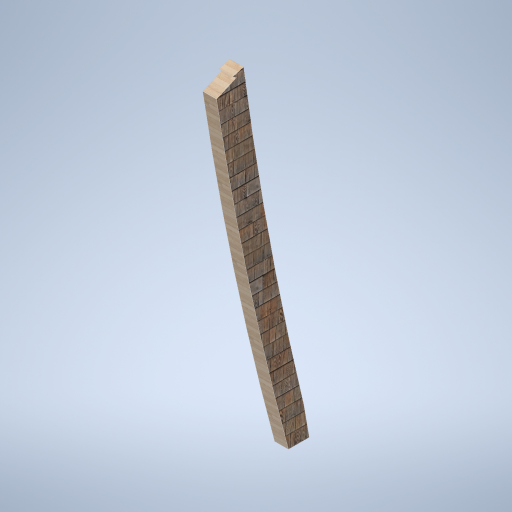
# Autodesk Inventor part: side_curve_beam_02
Saved by Autodesk Inventor 2024.2 (Build 282272000, 272)
## iProperties
Created: 2024-05-24
Part Number: side_curve_beam_02
Material: Wood (Maple)
Document SubType Name: Modeling
Designer: LOSTER_1
Density: 0.67 g/cm^3
Appearance: Natural Maple - Glossy Dark Tint
Author: LOSTER_1
Autodesk Inventor part; units mm, degrees
ref_plane "YZ Plane" through (0, 0, 0) normal (1, 0, 0) x (0, 1, 0)
ref_plane "XZ Plane" through (0, 0, 0) normal (0, 1, 0) x (-1, 0, 0)
ref_plane "XY Plane" through (0, 0, 0) normal (0, 0, 1) x (1, 0, 0)
sketch "Sketch1" plane through (0, 0, 0) normal (1, 0, 0) x (0, 1, 0)
  arc A0 (9232.7828, 59144.361) -> (9262.54, 59039.2764) centre (18869.1867, 61816.3864) ccw
  arc A1 (9080.0173, 59382.0678) -> (9192.4941, 59130.2744) centre (16896.114, 62722.5217) ccw
  arc A2 (9084.1758, 59429.1257) -> (9080.0173, 59382.0678) centre (9125.9944, 59401.7175) ccw
  ellipse E0 centre (9878.3873, 58718.5093) end of major axis (9878.3658, 59518.5093) minor radius 800 (9223.5152, 59178.0117) -> (9192.4941, 59130.2744) ccw
  arc A3 (9223.5152, 59178.0117) -> (9262.54, 59039.2764) centre (18869.1867, 61816.3864) ccw
  arc A4 (9262.54, 59039.2764) -> (5186.343, 58278.9896) centre (14548.8436, 19390.1277) ccw
  arc A5 (9080.0173, 59382.0678) -> (5136.0959, 58563.9551) centre (15222.25, 19856.4688) ccw
  line L0 (5186.343, 58278.9896) -> (4792.4199, 58209.5304)
  line L1 (4792.4199, 58209.5304) -> (4792.4199, 58472.769)
  arc A6 (5136.0959, 58563.9551) -> (4792.4199, 58472.769) centre (15222.25, 19856.4688) ccw
  point P0 (0, 0)
  point P1 (9076.1884, 59406.1188)
  point P2 (9232.7828, 59144.361)
  dimension "d0" = 40000
  dimension "d1" = 40000
  dimension "d2" = 400
  constraints: 15 point on circle, 7 centre point, 4 end point, 2 coincident, 1 vertical, 4 other
  measures "d0" radius of A4
  measures "d1" radius of A5
  measures "d2" distance of L0.start L0.end
extrude "Extrusion1" add sketch "Sketch1" along normal blind 175
body "Solid1"
